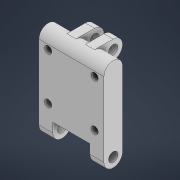
# Autodesk Inventor part: camera_arm
Saved by Autodesk Inventor 2021 (Build 250183000, 183)
## iProperties
Created: 2020-12-29
Part Number: camera_arm
Material: Generic
Document SubType Name: Modeling
Designer: Tomasz
Density: 1 g/cm^3
Appearance: Default
Author: Tomasz
Autodesk Inventor part; units mm, degrees
ref_plane "YZ Plane" through (0, 0, 0) normal (1, 0, 0) x (0, 1, 0)
ref_plane "XZ Plane" through (0, 0, 0) normal (0, 1, 0) x (-1, 0, 0)
ref_plane "XY Plane" through (0, 0, 0) normal (0, 0, 1) x (1, 0, 0)
sketch "Sketch1" plane through (0, 0, 0) normal (0, 0, 1) x (1, 0, 0)
  line L0 (0, 40) -> (0, 0)
  line L1 (0, 0) -> (6, 0)
  line L2 (6, 0) -> (6, 8)
  line L3 (6, 8) -> (22, 8)
  line L4 (22, 8) -> (22, 0)
  line L5 (22, 0) -> (28, 0)
  line L6 (28, 0) -> (28, 40)
  line L7 (28, 40) -> (0, 40)
  dimension "d0" = 6
  dimension "d1" = 6
  dimension "d2" = 16
  dimension "d3" = 40
  dimension "d4" = 8
  constraints: 16 end point, 7 perpendicular, 1 coincident, 1 horizontal alignment, 1 vertical
  measures "d0" distance between parallel lines of L2 L0
  measures "d1" distance between parallel lines of L4 L6
  measures "d2" distance of L2.end L3.end
  measures "d3" distance of L0.start L0.end
  measures "d4" distance of L1.end L2.end
extrude "Extrusion1" add sketch "Sketch1" against normal blind 8
sketch "Sketch2" plane through (28, 0, 0) normal (1, 0, 0) x (0, 0, -1)
  circle A0 centre (4, 4) radius 2
  line L0 (0, 0) -> (8, 0) projected
  line L1 (0, 0) -> (8, 0) projected
  point P0 (4, 0)
  dimension "d7" = 4
  dimension "d8" = 4
  dimension "d9" = 8
  constraints: 1 centre point, 1 midpoint, 1 vertical alignment
  measures "d7" diameter of A0
  measures "d8" distance from line of L0 A0.centre
  measures "d9" distance of L0.start L0.end
extrude "Extrusion2" cut sketch "Sketch2" against normal through all
fillet "Fillet1" radius 4 5 edges at (25, 0, 0) (3, 0, 0) (3, 0, -8) (25, 0, -8) (14, 8, -8)
sketch "Sketch3" plane through (0, 0, -8) normal (0, 0, -1) x (-1, 0, 0)
  line L0 (0, 40) -> (-28, 40) projected
  line L1 (-20, 40) -> (-16, 40)
  line L2 (-16, 40) -> (-16, 32)
  line L3 (-16, 32) -> (-20, 32)
  line L4 (-20, 32) -> (-20, 40)
  line L5 (-12, 40) -> (-8, 40)
  line L6 (-8, 40) -> (-8, 32)
  line L7 (-8, 32) -> (-12, 32)
  line L8 (-12, 32) -> (-12, 40)
  point P0 (0, 0)
  point P1 (-14, 40)
  dimension "d13" = 4
  dimension "d14" = 4
  dimension "d15" = 4
  dimension "d16" = 2
  dimension "d17" = 8
  constraints: 16 end point, 4 parallel, 2 horizontal, 2 perpendicular, 2 point on line, 1 horizontal alignment, 1 midpoint
  measures "d13" distance of L2.end L3.end
  measures "d14" distance of L6.end L7.end
  measures "d15" distance between parallel lines of L2 L8
  measures "d16" distance from line of point (-14, 40) L8
  measures "d17" distance of L3.end L1.start
extrude "Extrusion3" add sketch "Sketch3" along normal blind 8
sketch "Sketch4" plane through (20, 32, -8) normal (1, 0, 0) x (0, 0, -1)
  circle A0 centre (4, 4) radius 2
  line L0 (8, 8) -> (8, 0) projected
  point P0 (-8, -32)
  dimension "d20" = 4
  dimension "d21" = 8
  dimension "d22" = 4
  dimension "d23" = 4
  constraints: 1 centre point
  measures "d20" diameter of A0
  measures "d21" distance of L0.start L0.end
  measures "d22" distance from line of A0.centre L0
  measures "d23" horizontal distance of A0.centre L0.end
extrude "Extrusion4" cut sketch "Sketch4" against normal through all
fillet "Fillet2" radius 4 6 edges at (10, 40, -16) (18, 40, -16) (18, 32, -16) (10, 32, -16) (18, 32, -8) (10, 32, -8)
fillet "Fillet3" radius 4 4 edges at (14, 40, 0) (4, 40, -8) (14, 40, -8) (24, 40, -8)
sketch "Sketch5" plane through (0, 0, 0) normal (0, 0, 1) x (1, 0, 0)
  circle A0 centre (4, 34) radius 1.55
  line L0 (0, 36) -> (28, 36) construction
  line L1 (0, 36) -> (0, 4) construction
  circle A1 centre (4, 14) radius 1.55
  circle A2 centre (24, 34) radius 1.55
  circle A3 centre (24, 14) radius 1.55
  line L2 (28, 4) -> (28, 36) construction
  point P0 (0, 0)
  point P1 (14, 36)
  dimension "d30" = 20
  dimension "d33" = 20
  dimension "d36" = 2
  dimension "d37" = 10
  dimension "d38" = 3.1
  constraints: 4 centre point, 1 horizontal, 1 midpoint, 1 vertical, 6 other
  measures "d30" distance of A0.centre A1.centre
  measures "d33" distance of A0.centre A2.centre
  measures "d36" distance from line of L0 A0.centre
  measures "d37" horizontal distance of point (14, 36) A0.centre
  measures "d38" diameter of A0
extrude "Extrusion5" cut sketch "Sketch5" against normal up to surface (8 mm away)
equation "\"d0\" = d1"
equation "\"d4\" = 2 * arm_rod_diam"
equation "\"d5\" = 2 * arm_rod_diam"
equation "\"d7\" = arm_rod_diam"
equation "\"d8\" = 0.5 * d9"
equation "\"d12\" = arm_rod_diam"
equation "\"d13\" = d14"
equation "\"d16\" = 0.5 * d15"
equation "\"d18\" = 2 * arm_rod_diam"
equation "\"d20\" = arm_rod_diam"
equation "\"d22\" = 0.5 * d21"
equation "\"d23\" = d22"
equation "\"d26\" = arm_rod_diam"
equation "\"d27\" = arm_rod_diam"
equation "\"d37\" = 0.5 * d33"
equation "\"arm_rod_diam\" = 4"
body "Solid1"
